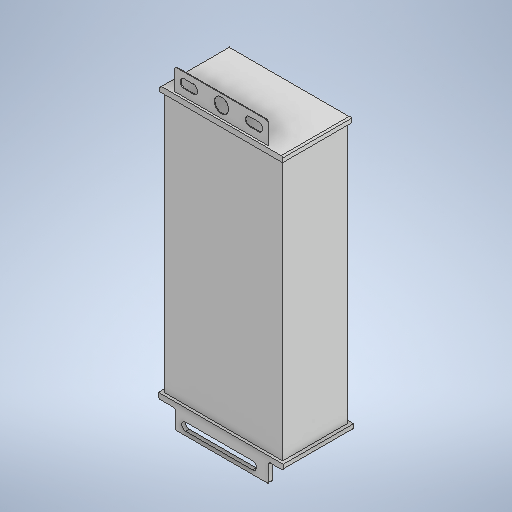
# Autodesk Inventor part: BLDC MOTORDRIVER
Saved by Autodesk Inventor 2025.2 (Build 292293000, 293)
## iProperties
Created: 2025-03-19
Part Number: BLDC MOTORDRIVER
Material: Generic
Document SubType Name: Modeling
Designer: Tobias
Density: 1 g/cm^3
Appearance: Default
Author: Tobias
Autodesk Inventor part; units mm, degrees
ref_plane "YZ Plane" through (0, 0, 0) normal (1, 0, 0) x (0, 1, 0)
ref_plane "XZ Plane" through (0, 0, 0) normal (0, 1, 0) x (-1, 0, 0)
ref_plane "XY Plane" through (0, 0, 0) normal (0, 0, 1) x (1, 0, 0)
sketch "Sketch1" plane through (0, 0, 0) normal (0, 1, 0) x (-1, 0, 0)
  line L0 (0, 0) -> (82, 0)
  line L1 (82, 0) -> (82, -45)
  line L2 (82, -45) -> (0, -45)
  line L3 (0, -45) -> (0, 0)
  dimension "d0" = 82
  dimension "d1" = 45
  constraints: 8 end point, 2 parallel, 1 horizontal, 1 perpendicular
  measures "d0" distance of L1.end L2.end
  measures "d1" distance of L0.end L1.end
extrude "Extrusion1" add sketch "Sketch1" along normal blind 188
sketch "Sketch2" plane through (0, 188, 0) normal (0, 1, 0) x (1, 0, 0)
  line L0 (0, 0) -> (-10, 0)
  line L1 (-82, 0) -> (0, 0) projected
  line L2 (-10, 0) -> (-75, 0)
  line L3 (-75, 0) -> (-75, 0.5)
  line L4 (-75, 0.5) -> (-10, 0.5)
  line L5 (-10, 0.5) -> (-10, 0)
  dimension "d4" = 10
  dimension "d5" = 65
  dimension "d6" = 0.5
  constraints: 10 end point, 2 parallel, 1 horizontal, 1 perpendicular, 1 point on line
  measures "d4" distance of L0.start L0.end
  measures "d5" distance of L3.end L4.end
  measures "d6" distance of L2.end L3.end
extrude "Extrusion2" add sketch "Sketch2" along normal blind 15
fillet "Fillet1" radius 2 2 edges at (-10, 203, -0.25) (-75, 203, -0.25)
sketch "Sketch3" plane through (-10, 188, -0.5) normal (0, 0, -1) x (-1, 0, 0)
  line L0 (0, 0) -> (-10, 0) projected
  line L1 (0, 0) -> (0, 8)
  line L2 (0, 0) -> (0, 13) projected
  line L3 (0, 8) -> (0, -24.5)
  line L4 (0, 8) -> (32.5, 8)
  circle A0 centre (32.5, 8) radius 5
  line L5 (32.5, 8) -> (55, 8)
  line L6 (55, 8) -> (10, 8)
  line L7 (49, 11) -> (61, 11)
  line L8 (61, 11) -> (61, 5)
  line L9 (61, 5) -> (49, 5)
  line L10 (49, 5) -> (49, 11)
  line L11 (49, 11) -> (61, 5) construction
  line L12 (61, 11) -> (49, 5) construction
  line L13 (4, 5) -> (16, 5)
  line L14 (16, 5) -> (16, 11)
  line L15 (16, 11) -> (4, 11)
  line L16 (4, 11) -> (4, 5)
  line L17 (4, 5) -> (16, 11) construction
  line L18 (16, 5) -> (4, 11) construction
  point P0 (-10, -188)
  dimension "d10" = 8
  dimension "d11" = 32.5
  dimension "d12" = 32.5
  dimension "d13" = 10
  dimension "d14" = 22.5
  dimension "d15" = 45
  dimension "d16" = 12
  dimension "d17" = 6
  dimension "d18" = 12
  dimension "d19" = 6
  constraints: 34 end point, 4 horizontal, 4 midpoint, 4 parallel, 3 point on line, 2 perpendicular, 1 centre point, 1 coincident
  measures "d10" distance of L0.start L1.end
  measures "d11" distance of L1.end L3.end
  measures "d12" distance of L1.end L4.end
  measures "d13" diameter of A0
  measures "d14" distance of L5.start L5.end
  measures "d15" distance of L5.end L6.end
  measures "d16" distance of L8.end L9.end
  measures "d17" distance of L7.end L8.end
  measures "d18" distance of L15.end L14.end
  measures "d19" distance of L14.end L13.end
extrude "Extrusion3" cut sketch "Sketch3" against normal blind 15
fillet "Fillet2" radius 3 4 edges at (-14, 193, -0.25) (-26, 193, -0.25) (-14, 199, -0.25) (-26, 199, -0.25)
fillet "Fillet3" radius 3 4 edges at (-71, 199, -0.25) (-71, 193, -0.25) (-59, 193, -0.25) (-59, 199, -0.25)
sketch "Sketch4" plane through (0, 188, 0) normal (0, 1, 0) x (1, 0, 0)
  line L0 (0, 0) -> (0, 45) projected
  line L1 (0, 0) -> (-82, 44.9424)
  line L2 (-82, 44.9424) -> (-82, 0)
  line L3 (0, 45) -> (-82, 45) projected
  line L4 (-82, 0) -> (0, 44.9424)
  line L5 (-83.5526, 46.5) -> (1.4474, 46.5)
  line L6 (1.4474, 46.5) -> (1.4474, -1.5)
  line L7 (1.4474, -1.5) -> (-83.5526, -1.5)
  line L8 (-83.5526, -1.5) -> (-83.5526, 46.5)
  line L9 (-83.5526, 46.5) -> (1.4474, -1.5) construction
  line L10 (1.4474, 46.5) -> (-83.5526, -1.5) construction
  point P0 (-41.0526, 22.5)
  dimension "d24" = 85
  dimension "d25" = 48
  constraints: 18 end point, 2 midpoint, 2 parallel, 2 perpendicular, 1 horizontal, 1 point on line
  measures "d24" distance of L6.end L7.end
  measures "d25" distance of L5.end L6.end
extrude "Extrusion4" add sketch "Sketch4" against normal blind 3.75 contours L1 L4 L0 | L4 L2 L1 | L5 L6 L7 L8
fillet "Fillet4" radius 1 3 edges at (-41.0526, 188, -46.5) (1.4474, 188, -22.5) (-83.5526, 188, -22.5)
sketch "Sketch5" plane through (0, 0, 0) normal (0, -1, 0) x (1, 0, 0)
  line L0 (-82, 0) -> (0, 0) projected
  line L1 (-82, -45) -> (-82, 0) projected
  line L2 (0, 0) -> (-82, -45)
  line L3 (0, 0) -> (0, -45) projected
  line L4 (-82, -45) -> (0, -45)
  line L5 (0, -45) -> (-82, 0)
  line L6 (2.25, -46.875) -> (-84.25, -46.875)
  line L7 (-84.25, -46.875) -> (-84.25, 1.875)
  line L8 (-84.25, 1.875) -> (2.25, 1.875)
  line L9 (2.25, 1.875) -> (2.25, -46.875)
  line L10 (2.25, -46.875) -> (-84.25, 1.875) construction
  line L11 (-84.25, -46.875) -> (2.25, 1.875) construction
  point P0 (-41, -22.5)
  dimension "d29" = 86.5
  dimension "d30" = 48.75
  constraints: 18 end point, 3 midpoint, 2 parallel, 2 perpendicular, 1 horizontal
  measures "d29" distance of L7.end L8.end
  measures "d30" distance of L6.end L7.end
extrude "Extrusion5" add sketch "Sketch5" against normal blind 3.75 contours L5 L2 L1 | L0 L2 L5 | L3 L5 L2 | L2 L5 L4 | L6 L7 L8 L9
fillet "Fillet5" radius 1 3 edges at (-41, 0, -46.875) (2.25, 0, -22.5) (-84.25, 0, -22.5)
sketch "Sketch6" plane through (0, 0, 0) normal (0, -1, 0) x (1, 0, 0)
  line L0 (2.25, 1.875) -> (2.25, -46.875) projected
  line L1 (2.25, 0) -> (-7.75, 0)
  line L2 (0, 0) -> (-82, 0) projected
  line L3 (-7.75, 0) -> (-7.75, 1.875)
  line L4 (-7.75, 1.875) -> (-72.75, 1.875)
  line L5 (-72.75, 1.875) -> (-72.75, -0.625)
  line L6 (-72.75, -0.625) -> (-7.75, -0.625)
  line L7 (-7.75, -0.625) -> (-7.75, 1.875)
  dimension "d34" = 10
  dimension "d35" = 65
  dimension "d36" = 2.5
  constraints: 12 end point, 2 parallel, 2 point on line, 1 horizontal, 1 perpendicular, 1 vertical
  measures "d34" distance of L1.start L1.end
  measures "d35" distance of L6.end L5.end
  measures "d36" distance of L5.end L4.end
extrude "Extrusion6" add sketch "Sketch6" along normal blind 13
fillet "Fillet6" radius 1 4 edges at (-72.75, -13, 0.625) (-72.75, 0, 0.625) (-7.75, -13, 0.625) (-7.75, 0, 0.625)
sketch "Sketch7" plane through (-84.25, 3.75, 1.875) normal (0, 0, 1) x (1, 0, 0)
  line L0 (75.5, -16.75) -> (12.5, -16.75) projected
  line L1 (56.3132, -16.75) -> (61.8132, -16.75)
  line L2 (65.2043, -16.75) -> (65.2043, -11.25)
  line L3 (65.2043, -11.25) -> (11.7642, -11.25)
  line L4 (65.2043, -11.25) -> (18.9706, -11.25) construction
  line L5 (65.2043, -8.5) -> (18.9706, -8.5)
  line L6 (18.9706, -14) -> (65.2043, -14)
  arc A0 (65.2043, -14) -> (65.2043, -8.5) centre (65.2043, -11.25) ccw
  arc A1 (18.9706, -8.5) -> (18.9706, -14) centre (18.9706, -11.25) ccw
  point P0 (84.25, -3.75)
  point P1 (42.0875, -11.25)
  dimension "d40" = 5.5
  dimension "d41" = 5.5
  constraints: 14 end point, 4 point on circle, 4 point on line, 4 tangent, 2 centre point, 1 midpoint, 1 parallel, 1 perpendicular, 1 vertical
  measures "d40" distance of L1.start L1.end
  measures "d41" distance of L2.start L2.end
extrude "Extrusion7" cut sketch "Sketch7" against normal blind 37.8
body "Solid1"
